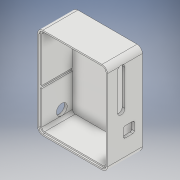
# Autodesk Inventor part: body
Saved by Autodesk Inventor 2019 (Build 230136000, 136)
## iProperties
Created: 2018-06-15
Part Number: body
Material: Generic
Document SubType Name: Modeling
Designer: daniel
Density: 1 g/cm^3
Appearance: Default
Author: daniel
Autodesk Inventor part; units mm, degrees
ref_plane "YZ Plane" through (0, 0, 0) normal (1, 0, 0) x (0, 1, 0)
ref_plane "XZ Plane" through (0, 0, 0) normal (0, 1, 0) x (-1, 0, 0)
ref_plane "XY Plane" through (0, 0, 0) normal (0, 0, 1) x (1, 0, 0)
sketch "Sketch3" plane through (0, 0, 0) normal (0, 0, 1) x (1, 0, 0)
  line L0 (-65, -85) -> (65, -85)
  line L1 (65, -85) -> (65, 85)
  line L2 (65, 85) -> (-65, 85)
  line L3 (-65, 85) -> (-65, -85)
  line L4 (-65, -85) -> (65, 85) construction
  line L5 (65, -85) -> (-65, 85) construction
  point P0 (0, 0)
  dimension "d7" = 130
  dimension "d8" = 170
  constraints: 12 end point, 2 midpoint, 2 parallel, 1 horizontal, 1 perpendicular
  measures "d7" distance of L2.end L1.end
  measures "d8" distance of L1.end L0.end
extrude "Extrusion3" add sketch "Sketch3" along normal blind 70
shell "Shell2" thickness 5 removed faces 1 at (21.6667, -28.3333, 70)
sketch "Sketch4" plane through (0, 0, 70) normal (0, 0, 1) x (1, 0, 0)
  line L0 (-91, 0) -> (91, 0) projected
  line L1 (0, 119) -> (0, -119) projected
  line L2 (-62.5, -13) -> (62.5, -13)
  line L3 (62.5, -13) -> (62.5, -8)
  line L4 (62.5, -8) -> (-62.5, -8)
  line L5 (-62.5, -8) -> (-62.5, -13)
  line L6 (-62.5, -13) -> (62.5, -8) construction
  line L7 (62.5, -13) -> (-62.5, -8) construction
  line L8 (-60, 80) -> (60, 80) projected
  line L9 (-65, 85) -> (-65, -85) projected
  point P0 (0, 0)
  point P1 (0, -10.5)
  dimension "d12" = 5
  dimension "d13" = 88
  dimension "d19" = 2.5
  constraints: 12 end point, 2 midpoint, 2 parallel, 1 horizontal, 1 perpendicular, 1 point on line
  measures "d12" distance of L3.end L2.end
  measures "d13" distance between parallel lines of L8 L4
  measures "d19" distance between parallel lines of L9 L5
extrude "Extrusion4" cut sketch "Sketch4" against normal up to surface (65 mm away)
sketch "Sketch8" plane through (65, -85, 0) normal (1, 0, 0) x (0, 0, -1)
  line L0 (-32.5, 81) -> (-46.5, 81)
  line L1 (-46.5, 81) -> (-46.5, 161)
  line L2 (-46.5, 161) -> (-32.5, 161)
  line L3 (-32.5, 161) -> (-32.5, 81)
  line L4 (-32.5, 81) -> (-46.5, 161) construction
  line L5 (-46.5, 81) -> (-32.5, 161) construction
  line L6 (0, 0) -> (0, 170) projected
  line L7 (-84, 85) -> (14, 85) projected
  point P0 (0, 85)
  point P1 (-39.5, 121)
  dimension "d42" = 32.5
  dimension "d43" = 80
  dimension "d44" = 14
  dimension "d66" = 36
  constraints: 12 end point, 2 parallel, 1 horizontal, 1 midpoint, 1 perpendicular
  measures "d42" distance between parallel lines of L6 L3
  measures "d43" distance of L0.end L1.end
  measures "d44" distance of L1.end L2.end
  measures "d66" distance from line of L7 point (-39.5, 121)
extrude "Extrusion6" cut sketch "Sketch8" against normal up to surface (5 mm away)
full round fillet "Fillet1" first side at (63.3333, 49.3333, 32.5) centre faces at (63.3333, -4, 37.1667) second side at (63.3333, 22.6667, 46.5)
full round fillet "Fillet2" first side at (63.3333, 51.6666, 32.5) centre faces at (63.3333, 76, 41.8333) second side at (63.3333, 27.3333, 46.5)
sketch "Sketch10" plane through (0, 0, 70) normal (0, 0, 1) x (1, 0, 0)
  line L0 (-65, -85) -> (65, -85)
  line L1 (65, -85) -> (65, 85)
  line L2 (65, 85) -> (-65, 85)
  line L3 (-65, 85) -> (-65, -85)
  line L4 (-65, -85) -> (65, 85) construction
  line L5 (65, -85) -> (-65, 85) construction
  point P0 (0, 0)
  dimension "d51" = 130
  dimension "d52" = 170
  constraints: 12 end point, 2 midpoint, 2 parallel, 1 horizontal, 1 perpendicular
  measures "d51" distance of L2.end L1.end
  measures "d52" distance of L1.end L0.end
extrude "Extrusion8" cut sketch "Sketch10" against normal blind 5
sketch "Sketch11" plane through (65, -85, 0) normal (1, 0, 0) x (0, 0, -1)
  line L0 (-15, 40) -> (-35, 40)
  line L1 (-35, 40) -> (-35, 60)
  line L2 (-35, 60) -> (-15, 60)
  line L3 (-15, 60) -> (-15, 40)
  line L4 (0, 0) -> (0, 170) projected
  line L5 (0, 0) -> (-70, 0) projected
  point P0 (0, 85)
  dimension "d59" = 15
  dimension "d60" = 40
  dimension "d63" = 20
  dimension "d64" = 20
  constraints: 8 end point, 2 parallel, 1 horizontal, 1 perpendicular
  measures "d59" distance between parallel lines of L4 L3
  measures "d60" distance between parallel lines of L5 L0
  measures "d63" distance of L0.start L0.end
  measures "d64" distance of L0.end L1.end
extrude "Extrusion9" cut sketch "Sketch11" against normal up to surface (5 mm away)
fillet "Fillet5" radius 3 4 edges at (62.5, -45, 15) (62.5, -25, 15) (62.5, -25, 35) (62.5, -45, 35)
sketch "Sketch12" plane through (0, 0, 65) normal (0, 0, 1) x (1, 0, 0)
  line L0 (62.5, 82.5) -> (-62.5, 82.5)
  line L1 (-62.5, 82.5) -> (-62.5, -82.5)
  line L2 (-62.5, -82.5) -> (62.5, -82.5)
  line L3 (62.5, -82.5) -> (62.5, 82.5)
  line L4 (62.5, 82.5) -> (-62.5, -82.5) construction
  line L5 (-62.5, 82.5) -> (62.5, -82.5) construction
  point P0 (0, 0)
  dimension "d68" = 125
  dimension "d69" = 165
  constraints: 12 end point, 2 midpoint, 2 parallel, 1 horizontal, 1 perpendicular
  measures "d68" distance of L2.end L1.end
  measures "d69" distance of L1.end L0.end
extrude "Extrusion10" cut sketch "Sketch12" against normal blind 3
fillet "Fillet6" radius 5 4 edges at (-60, -80, 33.5) (-60, 80, 33.5) (60, 80, 33.5) (60, -80, 33.5)
fillet "Fillet7" radius 7.5 4 edges at (-62.5, 82.5, 63.5) (-62.5, -82.5, 63.5) (62.5, 82.5, 63.5) (62.5, -82.5, 63.5)
fillet "Fillet4" radius 10 4 edges at (-65, -85, 32.5) (-65, 85, 32.5) (65, -85, 32.5) (65, 85, 32.5)
sketch "Sketch9" plane through (-65, -85, 0) normal (-1, 0, 0) x (0, 0, 1)
  circle A0 centre (25, 20) radius 10
  line L0 (0, 204) -> (0, -34) projected
  line L1 (-14, 85) -> (84, 85) projected
  point P0 (0, 85)
  dimension "d47" = 20
  dimension "d50" = 25
  dimension "d73" = 65
  constraints: 1 centre point
  measures "d47" diameter of A0
  measures "d50" distance from line of L0 A0.centre
  measures "d73" distance from line of L1 A0.centre
extrude "strombohrung" cut sketch "Sketch9" against normal up to surface (5 mm away)
body "Solid1"
body "Solid2"
